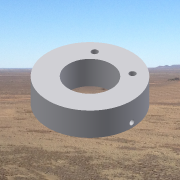
# Autodesk Inventor part: hub-cement
Saved by Autodesk Inventor 2013 (Build 170138000, 138)
## iProperties
Company: HERA Project
Created: 2013-05-20
Part Number: hub-cement
Material: Concrete
Document SubType Name: Modeling
Designer: David DeBoer
Density: 2.40731 g/cm^3
Description: Hub cement
Mass: 256229 g
Surface Area: 20937.4 cm^2
Volume: 106438 cm^3
Author: David DeBoer
Title: Cement
Autodesk Inventor part; units mm, degrees
ref_plane "YZ Plane" through (0, 0, 0) normal (1, 0, 0) x (0, 1, 0)
ref_plane "XZ Plane" through (0, 0, 0) normal (0, 1, 0) x (-1, 0, 0)
ref_plane "XY Plane" through (0, 0, 0) normal (0, 0, 1) x (1, 0, 0)
sketch "Sketch1" plane through (0, 0, 0) normal (0, 1, 0) x (-1, 0, 0)
  circle A0 centre (1.7415, 0) radius 450.85
  circle A1 centre (1.7415, 0) radius 229.87
  point P0 (0, 0)
  dimension "d0" = 901.7
  dimension "d4" = 459.74
  constraints: 2 centre point
  measures "d0" diameter of A0
  measures "d4" diameter of A1
extrude "Extrusion1" add sketch "Sketch1" along normal blind 254
sketch "Sketch2" plane through (-1.7415, 254, 0) normal (0, 1, 0) x (1, 0, 0)
  circle A0 centre (0, 0) radius 229.87 projected
  circle A1 centre (0, 0) radius 450.85 projected
  point P0 (1.7415, 0)
  point P1 (450.85, 0)
  constraints: 1 horizontal alignment, 1 other
ref_plane "Work Plane1" through (449.1085, 254, 0) normal (1, 0, 0) x (0, 1, 0)
sketch "Sketch3" plane through (449.1085, 254, 0) normal (1, 0, 0) x (0, 1, 0)
  circle A0 centre (-203.2, 0) radius 25.4
  line L0 (-254, 450.85) -> (-254, -450.85) projected
  point P0 (-254, 0)
  dimension "d5" = 50.8
  dimension "d6" = 50.8
  constraints: 1 centre point
  measures "d5" distance from line of A0.centre L0
  measures "d6" diameter of A0
extrude "Extrusion2" cut sketch "Sketch3" against normal blind 254
sketch "Sketch4" plane through (-1.7415, 254, 0) normal (0, 1, 0) x (1, 0, 0)
  circle A0 centre (0, 0) radius 229.87 projected
  circle A1 centre (0, 0) radius 450.85 projected
  circle A2 centre (-203.2, 254) radius 31.75
  circle A3 centre (1.7415, 0) radius 330.2 construction
  line L0 (0, 0) -> (0, 450.85) construction
  circle A4 centre (203.2, 254) radius 31.75
  dimension "d9" = 63.5
  dimension "d11" = 203.2
  dimension "d12" = 254
  constraints: 3 centre point, 2 end point, 1 symmetric about line, 1 vertical, 1 vertical alignment, 2 other
  measures "d9" diameter of A2
  measures "d11" horizontal distance of A2.centre A0.centre
  measures "d12" vertical distance of A0.centre A2.centre
extrude "Extrusion3" cut sketch "Sketch4" against normal blind 203.2 contours A2 | A4
body "Solid1"
